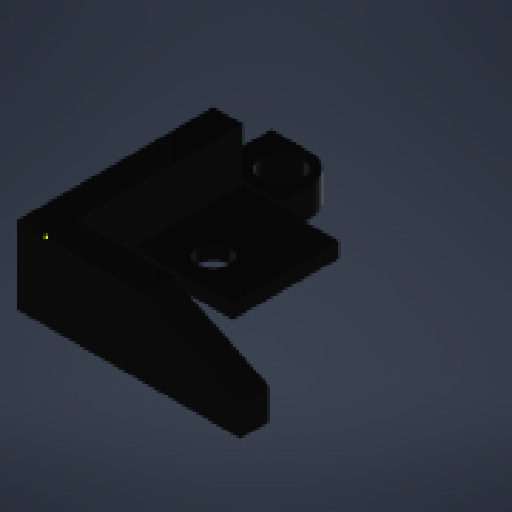
# Autodesk Inventor part: lfmw
Saved by Autodesk Inventor 2026.2 (Build 302298010, 298A)
## iProperties
Created: 2026-04-27
Part Number: lfmw
Material: Tworzywo sztuczne PET
Document SubType Name: Modeling
Designer: karol
Density: 1.541 g/cm^3
Appearance: Poliwęglan — przezroczysty
Mass: 0.888 g
Surface Area: 8.70622 cm^2
Volume: 0.888 cm^3
Author: karol
Autodesk Inventor part; units mm, degrees
ref_plane "YZ Plane" through (0, 0, 0) normal (1, 0, 0) x (0, 1, 0)
ref_plane "XZ Plane" through (0, 0, 0) normal (0, 1, 0) x (-1, 0, 0)
ref_plane "XY Plane" through (0, 0, 0) normal (0, 0, 1) x (1, 0, 0)
sketch "Szkic1" plane through (0, 0, 0) normal (0, 1, 0) x (-1, 0, 0)
  line L0 (0, 0) -> (3, 0)
  line L1 (3, 0) -> (3, -22)
  line L2 (3, -22) -> (0, -22)
  line L3 (0, -22) -> (0, 0)
  line L4 (0, 0) -> (-20, 0)
  line L5 (-20, 0) -> (-20, -3)
  line L6 (-20, -3) -> (0, -3)
  line L7 (0, -3) -> (0, 0)
  line L8 (0, -22) -> (-3, -22)
  line L9 (-3, -22) -> (-3, -17)
  line L10 (-3, -17) -> (0, -17)
  line L11 (0, -17) -> (0, -22)
  dimension "d0" = 3
  dimension "d1" = 22
  dimension "d2" = 20
  dimension "d3" = 3
  dimension "d4" = 3
  dimension "d5" = 5
  constraints: 24 end point, 6 parallel, 3 horizontal, 3 perpendicular
  measures "d0" distance of L1.end L2.end
  measures "d1" distance of L0.end L1.end
  measures "d2" distance of L6.end L5.end
  measures "d3" distance of L5.end L4.end
  measures "d4" distance of L9.end L10.end
  measures "d5" distance of L8.end L9.end
extrude "Wyciągnięcie proste1" add sketch "Szkic1" along normal blind 8
sketch "Szkic2" plane through (20, 0, -3) normal (0, 0, -1) x (-1, 0, 0)
  line L0 (0, 0) -> (0, 8) projected
  line L1 (0, 0) -> (20, 8)
  line L2 (23, 8) -> (0, 8) projected
  point P0 (20, 0)
  constraints: 2 end point, 1 point on line
extrude "Wyciągnięcie proste2" cut sketch "Szkic2" against normal blind 3
sketch "Szkic3" plane through (0, 8, 0) normal (0, 1, 0) x (1, 0, 0)
  point P0 (0, 0)
sketch "Szkic4" plane through (3, 0, -17) normal (1, 0, 0) x (0, 0, -1)
  line L0 (5, 0) -> (5, 8) projected
  line L1 (0, 0) -> (0, 8) projected
  line L2 (5, 0) -> (0, 0)
  line L3 (0, 0) -> (0, 8)
  line L4 (0, 8) -> (5, 8)
  line L5 (5, 8) -> (5, 0)
  point P0 (-17, 0)
  constraints: 8 end point, 2 parallel, 1 horizontal, 1 perpendicular
extrude "Wyciągnięcie proste3" cut sketch "Szkic4" against normal blind 3
sketch "Szkic5" plane through (0, 0, -22) normal (0, 0, -1) x (-1, 0, 0)
  line L0 (3, 8) -> (0, 8) projected
  line L1 (0, 0) -> (3, 0)
  line L2 (3, 0) -> (3, 8)
  line L3 (3, 8) -> (0, 8)
  line L4 (0, 8) -> (0, 0)
  constraints: 8 end point, 2 parallel, 1 horizontal, 1 perpendicular
extrude "Wyciągnięcie proste4" cut sketch "Szkic5" against normal blind 1.8
sketch "Szkic6" plane through (0, 0, -20.2) normal (0, 0, -1) x (-1, 0, 0)
  line L0 (3, 0) -> (3, 8) projected
  line L1 (3, 0) -> (-4, 0)
  line L2 (-4, 0) -> (-4, 3)
  line L3 (-4, 3) -> (3, 3)
  line L4 (3, 3) -> (3, 0)
  point P0 (0, 0)
  dimension "d14" = 7
  dimension "d15" = 3
  constraints: 8 end point, 2 parallel, 1 horizontal, 1 perpendicular
  measures "d14" distance of L2.end L3.end
  measures "d15" distance of L1.end L2.end
extrude "Wyciągnięcie proste5" add sketch "Szkic6" along normal blind 6
sketch "Szkic7" plane through (0, 3, -20.2) normal (0, 1, 0) x (1, 0, 0)
  circle A0 centre (1, 3) radius 2
  line L0 (-3, 0) -> (-3, 6) projected
  line L1 (-3, 6) -> (4, 6) projected
  point P0 (0, -20.2)
  point P1 (-3, 3)
  point P2 (0.5, 6)
  dimension "d18" = 4
  dimension "d19" = 4
  dimension "d20" = 3
  constraints: 2 midpoint, 1 centre point
  measures "d18" diameter of A0
  measures "d19" distance of point (-3, 3) A0.centre
  measures "d20" vertical distance of point (0.5, 6) A0.centre
extrude "Wyciągnięcie proste6" cut sketch "Szkic7" against normal blind 3
sketch "Szkic8" plane through (-3, 0, 0) normal (0, 0, 1) x (1, 0, 0)
  line L0 (3, 8) -> (13, 8)
  line L1 (23, 0) -> (3, 0) projected
  line L2 (23, 0) -> (23, 3.137)
  line L3 (13, 8) -> (23, 3.137)
  line L4 (23, 0) -> (3, 8) projected
  line L5 (3, 8) -> (23, 0)
  dimension "d23" = 10
  dimension "d24" = 3.137
  constraints: 8 end point, 1 collinear, 1 horizontal, 1 vertical
  measures "d23" distance of L0.start L0.end
  measures "d24" distance of L1.start L2.end
extrude "Wyciągnięcie proste7" add sketch "Szkic8" against normal blind 3
sketch "Szkic9" plane through (0, 0, -3) normal (1, 0, 0) x (0, 0, -1)
  line L0 (0, 0) -> (17.2, 0) projected
  line L1 (17.2, 0) -> (6.2, 0)
  line L2 (6.2, 0) -> (6.2, 1.5)
  line L3 (6.2, 1.5) -> (17.2, 1.5)
  line L4 (17.2, 1.5) -> (17.2, 0)
  point P0 (-3, 0)
  point P1 (6.2, 0)
  dimension "d27" = 11
  dimension "d35" = 1.5
  constraints: 8 end point, 2 parallel, 1 horizontal, 1 perpendicular
  measures "d27" distance of L2.end L3.end
  measures "d35" distance between parallel lines of L0 L3
extrude "Wyciągnięcie proste8" add sketch "Szkic9" along normal blind 10
sketch "Szkic10" plane through (0, 1.5, -9.2) normal (0, 1, 0) x (1, 0, 0)
  circle A0 centre (4.8, 3.2) radius 1.55
  line L0 (0, 0) -> (10, 0) projected
  line L1 (10, 11) -> (10, 0) projected
  line L2 (4, 11) -> (10, 11) projected
  line L3 (0, -6.2) -> (0, 11) projected
  point P0 (0, -9.2)
  point P1 (5, 0)
  dimension "d30" = 3.1
  dimension "d36" = 7.8
  dimension "d37" = 4.8
  constraints: 1 centre point, 1 midpoint
  measures "d30" diameter of A0
  measures "d36" distance from line of L2 A0.centre
  measures "d37" distance from line of L3 A0.centre
extrude "Wyciągnięcie proste9" cut sketch "Szkic10" against normal blind 2
fillet "Fillet1" radius 3 1 edges at (4, 1.5, -26.2)
sketch "Szkic11" plane through (0, 1.5, -9.2) normal (0, 1, 0) x (1, 0, 0)
  circle A0 centre (4.8, 3.2) radius 1.55 projected
  line L0 (0, 0) -> (0, 11) projected
  line L1 (0, 0) -> (10, 0) projected
  line L2 (10, 11) -> (10, 0) projected
  line L3 (4, 11) -> (10, 11) projected
  line L4 (0, 11) -> (4, 11) projected
  point P0 (0, -9.2)
extrude "Wyciągnięcie proste10" add sketch "Szkic11" along normal blind 1
sketch "Szkic12" plane through (0, 0, 0) normal (0, -1, 0) x (1, 0, 0)
  line L0 (10, -9.2) -> (10, -20.2) projected
  line L1 (10, -20.2) -> (4, -20.2) projected
  line L2 (0, -20.2) -> (4, -20.2) projected
  line L3 (0, -9.2) -> (0, -20.2) projected
  line L4 (0, -9.2) -> (10, -9.2) projected
  circle A0 centre (4.8, -12.4) radius 1.55 projected
  point P0 (0, 0)
extrude "Wyciągnięcie proste11" cut sketch "Szkic12" against normal blind 1
